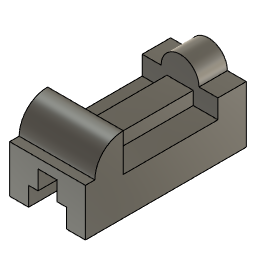
f2 v1 (Autodesk Fusion 360 design; units mm, degrees)
Autodesk Fusion 360 part; units mm, degrees
sketch "Sketch1" plane through (0, 0, 0) normal (0, 0, 1) x (1, 0, 0)
  line L0 (0, 0) -> (80, 0)
  line L1 (80, 0) -> (80, 170)
  line L2 (80, 170) -> (0, 170)
  line L3 (0, 170) -> (0, 0)
  dimension "d1" = 80
  dimension "d2" = 170
  constraint horizontal L0
  constraint vertical L1
  constraint horizontal L2
  constraint vertical L3
  constraint coincident L0.start L3.end
  measures "d1" distance of L0.start L0.end
  measures "d2" distance of L0.start L2.end
extrude "Extrude1" add sketch "Sketch1" along normal blind 80
sketch "Sketch2" plane through (80, 0, 0) normal (1, 0, 0) x (0, 1, 0)
  line L0 (0, 0) -> (170, 0)
  line L1 (170, 0) -> (170, 80)
  line L2 (170, 80) -> (0, 80)
  line L3 (0, 80) -> (0, 0)
  line L4 (0, 50) -> (10, 50)
  arc A0 (40, 80) -> (10, 50) centre (40, 50) ccw
  line L5 (40, 80) -> (40, 40)
  line L6 (40, 40) -> (140, 40)
  line L7 (140, 40) -> (140, 60)
  line L8 (140, 60) -> (170, 60)
  dimension "d5" = 10
  dimension "d6" = 30
  dimension "d8" = 40
  dimension "d9" = 30
  dimension "d10" = 20
  dimension "d12" = 30
  constraint coincident L3 L4.start
  constraint perpendicular L3 L4
  constraint coincident L2 A0.start
  constraint perpendicular L2 L5
  constraint vertical A0.centre L5.end
  constraint perpendicular L5 L6
  constraint perpendicular L2 L7
  constraint coincident L1 L8.end
  constraint perpendicular L1 L8
  measures "d5" distance of L4.start L4.end
  measures "d6" distance of L2 L4
  measures "d8" distance of A0.start L5.end
  measures "d9" distance of L4.end A0.centre
  measures "d10" distance of L6.end L7.end
  measures "d12" distance of L7.end L8.end
extrude "Extrude2" cut sketch "Sketch2" against normal blind 80 contours L2 L3 L4 A0 | L1 L2 L5 L6 L7 L8
sketch "Sketch3" plane through (0, 170, 0) normal (0, 1, 0) x (-1, 0, 0)
  line L0 (0, 60) -> (-80, 60)
  line L1 (-80, 60) -> (-80, 0)
  line L2 (-80, 0) -> (0, 0)
  line L3 (0, 0) -> (0, 60)
  arc A0 (-20, 60) -> (-60, 60) centre (-40, 60) ccw
  dimension "d15" = 20
  constraint coincident L0 A0.end
  constraint midpoint L0 A0.centre
  measures "d15" radius of A0
extrude "Extrude3" add sketch "Sketch3" against normal blind 30 contours L0 A0
sketch "Sketch4" plane through (0, 0, 0) normal (0, -1, 0) x (1, 0, 0)
  line L0 (80, 50) -> (0, 50)
  line L1 (0, 50) -> (0, 0)
  line L2 (0, 0) -> (80, 0)
  line L3 (80, 0) -> (80, 50)
  line L4 (40, 50) -> (40, -1.5381) construction
  line L5 (20, 0) -> (20, 20)
  line L6 (20, 20) -> (30, 20)
  line L7 (30, 20) -> (30, 40)
  line L8 (30, 40) -> (40, 40)
  line L9 (60, 0) -> (60, 20)
  line L10 (50, 40) -> (40, 40)
  line L11 (60, 20) -> (50, 20)
  line L12 (50, 20) -> (50, 40)
  dimension "d18" = 20
  dimension "d19" = 10
  dimension "d20" = 20
  dimension "d21" = 10
  constraint midpoint L0 L4.start
  constraint perpendicular L2 L4
  constraint coincident L2 L5.start
  constraint perpendicular L2 L5
  constraint perpendicular L5 L6
  constraint perpendicular L2 L7
  constraint coincident L4 L8.end
  constraint perpendicular L4 L8
  constraint symmetric L4 L5.start L9.start
  constraint symmetric L4 L5.end L9.end
  constraint symmetric L4 L6.end L11.end
  constraint symmetric L4 L7.end L10.start
  constraint symmetric L4 L8.end L10.end
  measures "d18" distance of L1 L5
  measures "d19" distance of L5.end L6.end
  measures "d20" distance of L5.start L5.end
  measures "d21" distance of L0 L8
extrude "Extrude4" cut sketch "Sketch4" against normal blind 170 contours L2 L5 L6 L7 L8 L9 L10 L11 L12
sketch "Sketch5" plane through (0, 40, 0) normal (0, 1, 0) x (-1, 0, 0)
  line L0 (-80, 80) -> (-80, 40)
  line L1 (-80, 40) -> (-50, 40)
  line L2 (-50, 40) -> (-30, 40)
  line L3 (-30, 40) -> (0, 40)
  line L4 (0, 40) -> (0, 80)
  line L5 (0, 80) -> (-80, 80)
  line L6 (-50, 40) -> (-50, 50)
  line L7 (-50, 50) -> (-30, 50)
  line L8 (-30, 40) -> (-30, 42.318)
  line L9 (-30, 42.318) -> (-30, 50)
  line L10 (-53.8731, 40) -> (-53.8731, 53.8731)
  line L11 (-53.8731, 53.8731) -> (-26.1269, 53.8731)
  line L12 (-26.1269, 42.318) -> (-26.1269, 53.8731)
  line L13 (-26.1269, 40) -> (-26.1269, 42.318)
  dimension "d24" = 10
  dimension "d25" = -3.8731
  constraint coincident L1.end L2.start
  constraint perpendicular L1 L6
  constraint perpendicular L6 L7
  constraint coincident L2.end L3.start
  constraint perpendicular L3 L8
  constraint perpendicular L7 L9
  measures "d24" distance of L1.end L6.end
extrude "Extrude5" add sketch "Sketch5" along normal blind 100 contours L1 L3 L6 L7 L8 L9 L10 L11 L12 L13
